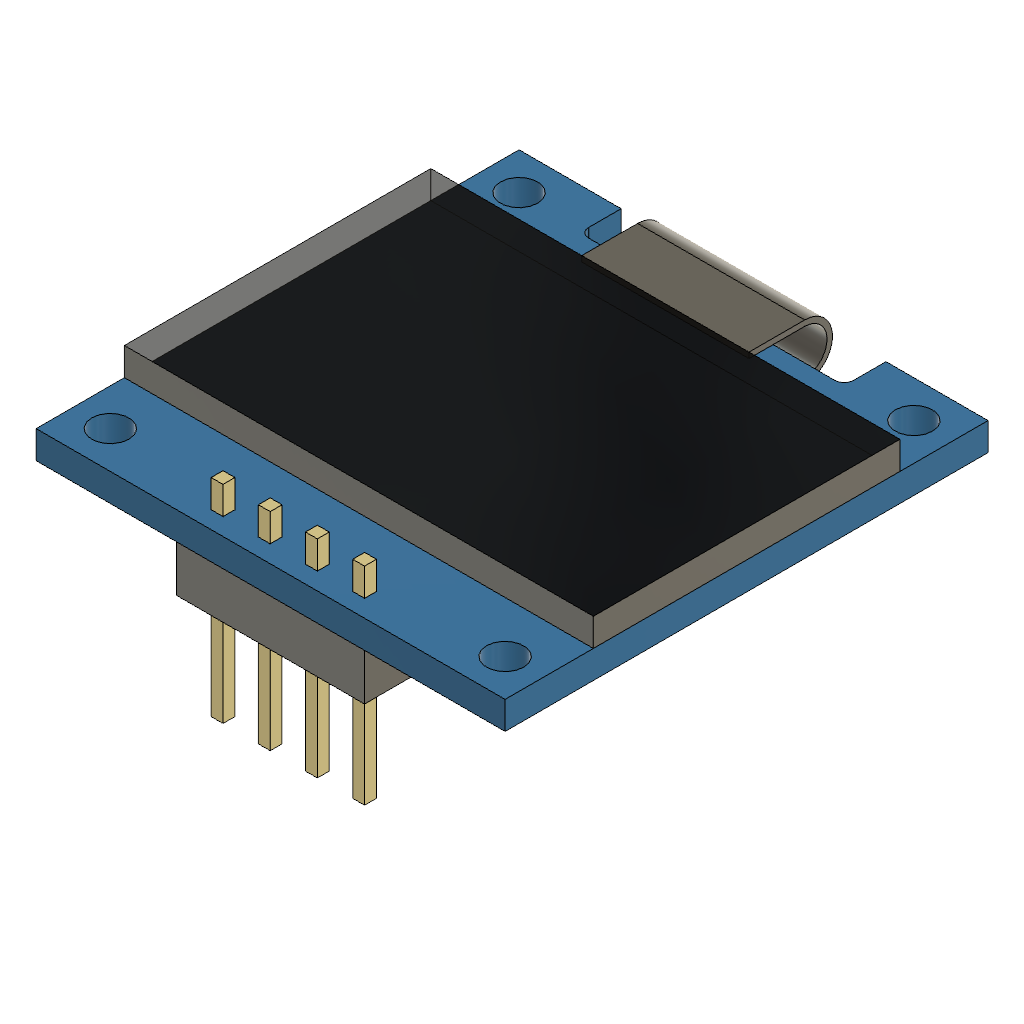
Case_Oled_Screen (Autodesk Fusion 360 archive; units mm, degrees)
design "SSD1306_OLED_0.96in"
description: Open CASCADE Model
Autodesk Fusion 360 part; units mm, degrees
sketch "Sketch1" plane through (0, 0, 0) normal (0, 0, 1) x (1, 0, 0)
  line L0 (-12.625, 13) -> (-7.125, 13)
  line L1 (-7.125, 13) -> (-7.125, 11.25)
  arc A0 (-7.125, 11.25) -> (-6.625, 10.75) centre (-6.625, 11.25) ccw
  line L2 (-6.625, 10.75) -> (6.625, 10.75)
  arc A1 (6.625, 10.75) -> (7.125, 11.25) centre (6.625, 11.25) ccw
  line L3 (7.125, 11.25) -> (7.125, 13)
  line L4 (7.125, 13) -> (12.625, 13)
  line L5 (12.625, 13) -> (12.625, -13)
  line L6 (12.625, -13) -> (-12.625, -13)
  line L7 (-12.625, -13) -> (-12.625, 13)
  circle A2 centre (-10.625, 11) radius 1
  circle A3 centre (10.625, 11) radius 1
  circle A4 centre (10.625, -11) radius 1
  circle A5 centre (-10.625, -11) radius 1
  line L8 (-4.13, -11.43) -> (-3.49, -11.43)
  line L9 (-3.49, -11.43) -> (-3.49, -12.07)
  line L10 (-3.49, -12.07) -> (-4.13, -12.07)
  line L11 (-4.13, -12.07) -> (-4.13, -11.43)
  line L12 (-5.06, -10.5) -> (5.06, -10.5)
  line L13 (5.06, -10.5) -> (5.06, -13)
  line L14 (5.06, -13) -> (-5.06, -13)
  line L15 (-5.06, -13) -> (-5.06, -10.5)
  line L16 (-4.13, -11.43) -> (-5.06, -10.5) construction
  line L17 (-1.59, -12.07) -> (-1.59, -11.43)
  line L18 (-1.59, -11.43) -> (-0.95, -11.43)
  line L19 (-0.95, -12.07) -> (-1.59, -12.07)
  line L20 (-0.95, -11.43) -> (-0.95, -12.07)
  line L21 (0.95, -12.07) -> (0.95, -11.43)
  line L22 (0.95, -11.43) -> (1.59, -11.43)
  line L23 (1.59, -12.07) -> (0.95, -12.07)
  line L24 (1.59, -11.43) -> (1.59, -12.07)
  line L25 (3.49, -12.07) -> (3.49, -11.43)
  line L26 (3.49, -11.43) -> (4.13, -11.43)
  line L27 (4.13, -12.07) -> (3.49, -12.07)
  line L28 (4.13, -11.43) -> (4.13, -12.07)
  line L29 (4.13, -11.43) -> (5.06, -10.5) construction
  line L30 (-0.95, -11.75) -> (0.95, -11.75) construction
  line L31 (-12.625, 8.25) -> (12.625, 8.25)
  line L32 (12.625, 8.25) -> (12.625, -8.25)
  line L33 (12.625, -8.25) -> (-12.625, -8.25)
  line L34 (-12.625, -8.25) -> (-12.625, 8.25)
  line L35 (-4.5, 12.75) -> (4.5, 12.75)
  line L36 (4.5, 12.75) -> (4.5, 8.25)
  line L37 (4.5, 8.25) -> (-4.5, 8.25)
  line L38 (-4.5, 8.25) -> (-4.5, 12.75)
  line L39 (-12.625, 5.25) -> (12.625, 5.25)
  point P0 (-12.625, 0)
  point P1 (0, -13)
  point P2 (-4.13, -11.75)
  point P3 (-5.06, -11.75)
  point P4 (0, -11.75)
  point P5 (0, 12.75)
  dimension "d1" = 25.25
  dimension "d2" = 26
  dimension "d3" = 2.25
  dimension "d4" = 0.5
  dimension "d5" = 5.5
  dimension "d6" = 45
  dimension "d7" = 0.64
  dimension "d10" = 2.54
  dimension "d11" = 0
  dimension "d12" = 2.5
  dimension "d13" = 2
  dimension "d14" = 2
  dimension "d15" = 2
  dimension "d16" = 2
  dimension "d17" = 2
  dimension "d18" = 4.75
  dimension "d19" = 4.75
  dimension "d20" = 0.25
  dimension "d21" = 9
  dimension "d39" = 3
  constraint horizontal L0
  constraint perpendicular L0 L1
  constraint tangent L1 A0
  constraint tangent L2 A1
  constraint perpendicular L0 L3
  constraint tangent A0 L2
  constraint tangent A1 L3
  constraint horizontal L4
  constraint horizontal L6
  constraint perpendicular L5 L6
  constraint perpendicular L6 L7
  constraint perpendicular L1 L2
  constraint equal L0 L4
  constraint midpoint L7 P0
  constraint horizontal origin P0
  constraint midpoint L6 P1
  constraint vertical origin P1
  constraint equal L5 L7
  constraint horizontal L8
  constraint vertical L9
  constraint horizontal L10
  constraint vertical L11
  constraint horizontal L12
  constraint vertical L13
  constraint horizontal L14
  constraint vertical L15
  constraint coincident L6 L13.end
  constraint equal L8 L9
  constraint midpoint L11 P2
  constraint midpoint L15 P3
  constraint horizontal P2 P3
  constraint perpendicular L16 L29
  constraint midpoint L20 L30.start
  constraint midpoint L21 L30.end
  constraint midpoint L30 P4
  constraint vertical origin P4
  constraint equal A2 A5
  constraint equal A0 A1
  constraint equal A3 A4
  constraint equal A4 A5
  constraint vertical A2.centre A5.centre
  constraint horizontal A4.centre A5.centre
  constraint vertical A3.centre A4.centre
  constraint horizontal A2.centre A3.centre
  constraint horizontal L31
  constraint vertical L32
  constraint horizontal L33
  constraint vertical L34
  constraint coincident L5 L32.end
  constraint coincident L7 L31.start
  constraint horizontal L35
  constraint vertical L36
  constraint horizontal L37
  constraint vertical L38
  constraint coincident L31 L36.end
  constraint midpoint L35 P5
  constraint vertical origin P5
  constraint coincident L34 L39.start
  constraint coincident L32 L39.end
  constraint horizontal L39
  measures "d1" distance of L5.end L6.end
  measures "d2" distance of L4 L6
  measures "d3" distance of L2 L4
  measures "d4" radius of A1
  measures "d5" distance of L3.end L4.end
  measures "d6" angle of L12 L16
  measures "d7" distance of L8.start L8.end
  measures "d12" distance of L12.start L14.end
  measures "d13" diameter of A5
  measures "d14" distance of L0 A2.centre
  measures "d15" distance of L7 A2.centre
  measures "d16" distance of L6 A4.centre
  measures "d17" distance of L5 A4.centre
  measures "d18" distance of L4 L31
  measures "d19" distance of L6 L33
  measures "d20" distance of L4 L35
  measures "d21" distance of L35.start L35.end
  measures "d39" distance of L31 L39
extrude "Extrude1" add sketch "Sketch1" against normal blind 1.5 contours L0 L1 A0 L2 L7 L31 L38 | L5 L7 L31 L32 L34 L37 L39 | L5 L7 L32 L33 L34 L39 | L2 L31 L36 L37 L38 | L5 L6 L7 L12 L13 L15 L33 | L2 A1 L3 L4 L5 L31 L36 | L6 L12 L13 L14 L15 makes body 1
extrude "Extrude2" add sketch "Sketch1" along normal blind 1.5 separate body contours L5 L7 L31 L32 L34 L37 L39 | L5 L7 L32 L33 L34 L39 makes body 2
extrude "Extrude3" add sketch "Sketch1" along normal mid plane 3 separate body contours L2 L31 L36 L37 L38 | L2 L35 L36 L38 makes body 3
shell "Shell1" thickness 0.3 removed faces 3 at (-4.5, 11.25, 0.5) at (4.5, 11.25, -0.5) at (1.5, 8.25, 0.5) on bodies 3
extrude "Extrude4" add sketch "Sketch1" against normal blind 11.15 from surface at 1.5 separate body contours L8 L9 L10 L11 | L17 L18 L19 L20 | L21 L22 L23 L24 | L25 L26 L27 L28 makes body 4 at (-1.59, -11.8567, -5.9333) makes body 5 at (0.95, -11.8567, -5.9333) makes body 6 at (-3.49, -11.6433, -5.9333) makes body 7 at (3.49, -11.8567, -5.9333)
extrude "Extrude5" add sketch "Sketch1" against normal blind 2.5 from surface at -1.5 separate body contours L6 L12 L13 L14 L15 makes body 8
fillet "Fillet1" radius 1.5 2 edges at (0, 12.75, 1.5) (0, 12.75, -1.5) on bodies 3
fillet "Fillet1" radius 1.2 2 edges at (0, 12.45, 1.2) (0, 12.45, -1.2) on bodies 3
equation "d15 = d14"
equation "d16 = d14"
equation "d17 = d16"
equation "d19 = d18"
